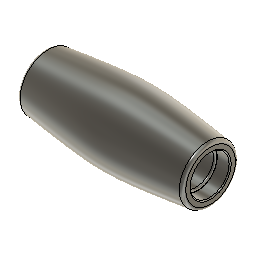
18650 Rotator handle v4 (Autodesk Fusion 360 design; units mm, degrees)
Autodesk Fusion 360 part; units mm, degrees
note: some values were not read from the file. Chosen so that the rebuilt part matches the saved one: which face or edge a step refers to. Set by a fixed rule: which sketch regions a step uses.
sketch "handle" plane through (0, 0, 0) normal (0, 0, 1) x (1, 0, 0)
  line L0 (6.0662, 10) -> (6.0662, 11.2)
  line L1 (-1.3338, 11.2) -> (-1.3338, 16)
  line L2 (86.2662, 10) -> (86.2662, 11.2)
  line L3 (86.2662, 11.2) -> (93.6662, 11.2)
  line L4 (93.6662, 11.2) -> (93.6662, 16)
  spline S0 degree 5 poles (-1.3338, 16) (4.5165, 16.7313) (15.1706, 18.0263) (28.0147, 19.4663) (40.1009, 20.4822) (52.2314, 20.4822) (64.3176, 19.4663) (77.1617, 18.0263) (87.8158, 16.7313) (93.6662, 16) knots 0 0 0 0 0 0 0.2 0.4 0.6 0.8 1 1 1 1 1 1
  line L5 (-9.3338, 15) -> (6.6662, 17)
  line L6 (85.6662, 17) -> (101.6662, 15)
  line L7 (6.0662, 10) -> (86.2662, 10)
  line L8 (6.0662, 11.2) -> (-1.3338, 11.2)
  line L9 (0, 0) -> (94, 0)
  dimension "d8" = 95
  dimension "d9" = 7.4
  dimension "d10" = 7.4
  dimension "d11" = 11.2
  dimension "d13" = 10
  dimension "d14" = 16
  dimension "d15" = 16
  dimension "d16" = 11.2
  dimension "d17" = 8
  dimension "d18" = 8
  dimension "d19" = 15
  dimension "d20" = 15
  constraint vertical L0
  constraint perpendicular L2 L3
  constraint perpendicular L3 L4
  constraint midpoint L1.end L5
  constraint midpoint L4.end L6
  constraint perpendicular L1 L8
  constraint coincident L9.start origin
  constraint parallel L7 L9
  constraint horizontal L9
  constraint parallel L8 L9
  measures "d8" distance of L1 L4
  measures "d9" distance of L2.end L3.end
  measures "d10" distance of L0.end L1.start
  measures "d11" distance of L9.start L3
  measures "d13" distance of L9.start L7
  measures "d14" vertical distance of L9.start L1.end
  measures "d15" vertical distance of L9.start L4.end
  measures "d16" vertical distance of L9.start L1.start
  measures "d17" horizontal distance of L1.end L5.start
  measures "d18" horizontal distance of L4.end L6.end
  measures "d19" distance of L6.end L9
  measures "d20" vertical distance of L9.start L5.start
revolve "Revolve1" add sketch "handle" angle 360 about axis through (1.75, 0, 0) along (1, 0, 0)
fillet "Fillet1" radius 1 2 edges at (6.0662, -3.6162, 9.3233) (86.2662, -3.6162, 9.3233)
fillet "Fillet2" radius 0.6 1 edges at (93.6662, -11.2, 0)
fillet "Fillet3" radius 2 2 edges at (-1.3338, -5.7858, 14.9172) (93.6662, -5.7858, 14.9172)
named bodies: "RotatorHandle"
